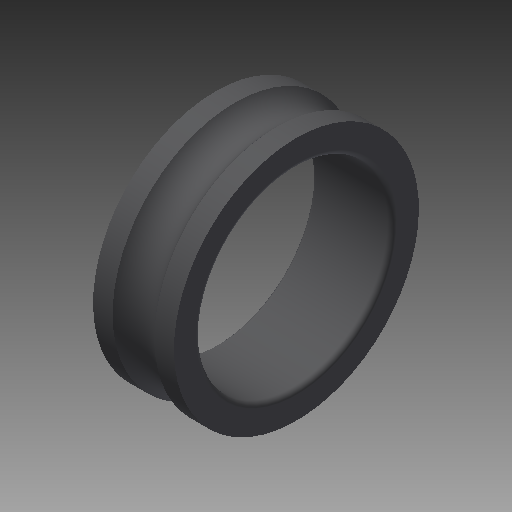
# Autodesk Inventor part: 6209_PART1
Saved by Autodesk Inventor 2018 (Build 220112000, 112)
## iProperties
Category: PARTsolutions
Company: SKF
Created: 2018-05-06
Part Number: 6209_PART1
Catalog Web Link: www.cadenas.de
Description: -Deep groove ball bearings, single row
Vendor: SKF
Document SubType Name: Modeling
Designer: psAdmin
Manufacturer: SKF
Mass: 16.2761 g
Surface Area: 81.8903 cm^2
Volume: 16.2761 cm^3
Density: 1 g/cm^3
Material: Generic
Appearance: PSOLRGB-175-175-175
PSOL_IDENT_0: {$CADENAS_DATA\23d-libs\skf\bearings_units_and_housings\ball_bearings\deep_groove_ball_bearings\deep
PSOL_IDENT_1: _groove_ball_bearings_single_row\bb1_001_101.prj},190 {VTYP=3D},{NB=6209_PART1},{LINA=6209_PART1},{N
PSOL_IDENT_2: N=BB1_001_101_PART1},{NOPRJ=TRUE},{DATE=14.07.2017 09:01:20},{GEOMDATE=14.07.2017 08:21:21},{VERSION=
PSOL_IDENT_3: },{LINEID=216350},{LINESUBID=-1},{WBVAR=}  {NB=6209_PART1},{LINA=6209_PART1},{KT=DUMMY},{PRODUCTID=1
PSOL_IDENT_4: 050010209},{DESIGNATION=6209},{DD=45.000},{D=85.000},{B=19.000},{HH=-1000000015047466219876688855040
PSOL_IDENT_5: .000},{DD1=57.600},{DD2=-1000000015047466219876688855040.000},{DD22=-1000000015047466219876688855040
PSOL_IDENT_6: .000},{D1=72.400},{D2=75.190},{BB=-1000000015047466219876688855040.000},{R12=1.1},{R121=1.100},{R122=
PSOL_IDENT_7: 1.000},{LOAD1=35.100},{LOAD2=21.600},{LOAD3=0.915},{SPEED1=17000},{SPEED2=11000},{MASS=0.416},{PITCH=
PSOL_IDENT_8: 65.000},{DW=12.303},{Z=10.000},{II=1.000},{TYPEID=105001},{HELP=6.3},{HELP2=4.905},{DD1ALG=28.8},{TA
PSOL_IDENT_9: XONOMY=1},{DESIGN=dgbb1},{MAPPING=BCZ50,DESIGNATION|IRD01,DD|ORD10,D|BCW30,B|ORL64,HH|IRD30,DD1|IRD4
PSOL_IDENT_10: 6,DD2|IRD43,DD22|ORD30,D1|ORD43,D2|ORL60,BB|ORL03,R121|BCE41,R122|BCC02,LOAD1|BCC16,LOAD2|BCC12,LOAD
PSOL_IDENT_11: 3|BCC43,SPEED1|BCC45,SPEED2|BCM01,MASS|BCD50,PITCH|RBD10,DW|BCN81,Z|BCN80,II},{DESIGNLIST=dgbbrs,dgb
PSOL_IDENT_12: b1,dgbb2rs,dgbb2z,dgbbn1,dgbbz},{YALG=28.80000},{HALG=6.30000},{YALG1=36.20000},{HALG1=6.30000},{PIT
PSOL_IDENT_13: CH1=65.00000},{DW1=12.30300},{SH=28.8},{CU=1.3394},{SORT=DD},{PIM=6209}
NT: Deep groove ball bearings, single row
NB: 6209_PART1
NBSYN: $DESIGNATION._PART1
LINA: 6209_PART1
DESIGNATION: 6209
DD: 45.000
D: 85.000
B: 19.000
LOAD1: 35.100
LOAD2: 21.600
LOAD3: 0.915
SPEED1: 17000
SPEED2: 11000
SUPPLIER: SKF
ARTICLENO: 6209_PART1
BOMINFO: 6209_PART1
CREATOR: CADENAS GmbH
Title: 6209_PART1
Author: Cadenas PARTsolutions
Comments: Deep groove ball bearings, single row
Autodesk Inventor part; units mm, degrees
ref_plane "YZ Plane" through (0, 0, 0) normal (1, 0, 0) x (0, 1, 0)
ref_plane "XZ Plane" through (0, 0, 0) normal (0, 1, 0) x (-1, 0, 0)
ref_plane "XY Plane" through (0, 0, 0) normal (0, 0, 1) x (1, 0, 0)
sketch "Sketch_1" plane through (0, 0, 0) normal (0, 0, 1) x (1, 0, 0)
  line L0 (50, 0) -> (-50, 0)
  arc A0 (0, 23.6) -> (1.1, 22.5) centre (1.1, 23.6) ccw
  line L1 (1.1, 22.5) -> (17.9, 22.5)
  arc A1 (17.9, 22.5) -> (19, 23.6) centre (17.9, 23.6) ccw
  line L2 (19, 23.6) -> (19, 28.8)
  line L3 (19, 28.8) -> (14.4144, 28.8)
  arc A2 (4.5856, 28.8) -> (14.4144, 28.8) centre (9.5, 32.5) ccw
  line L4 (4.5856, 28.8) -> (0, 28.8)
  line L5 (0, 28.8) -> (0, 23.6)
  constraints: 12 end point, 6 point on circle, 3 centre point
revolve "Revolution1" add sketch "Sketch_1" angle 360 about axis through (50, 0, 0) along (1, 0, 0)
body "Solid1"
